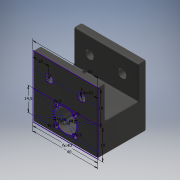
# Autodesk Inventor part: z_nut_holder
Saved by Autodesk Inventor 2018 (Build 220112000, 112)
## iProperties
Created: 2018-05-29
Part Number: z_nut_holder
Material: ABS Plastic
Document SubType Name: Modeling
Designer: Z. Deniz
Density: 1.06 g/cm^3
Appearance: Smooth - White
Author: Z. Deniz
Autodesk Inventor part; units mm, degrees
ref_plane "YZ Plane" through (0, 0, 0) normal (1, 0, 0) x (0, 1, 0)
ref_plane "XZ Plane" through (0, 0, 0) normal (0, 1, 0) x (-1, 0, 0)
ref_plane "XY Plane" through (0, 0, 0) normal (0, 0, 1) x (1, 0, 0)
sketch "Sketch1" plane through (0, 0, 0) normal (0, 1, 0) x (-1, 0, 0)
  circle A0 centre (0, 0) radius 7
  circle A1 centre (0, 0) radius 8 construction
  line L0 (0, 0) -> (5.6569, -5.6569) construction
  line L1 (0, 0) -> (8, 0) construction
  line L2 (0, 0) -> (-5.6569, -5.6569) construction
  line L3 (0, 0) -> (8, 0) construction
  line L4 (0, 0) -> (5.6569, 5.6569) construction
  line L5 (0, 0) -> (-5.6569, 5.6569) construction
  arc A2 (5.6319, 4.1571) -> (4.1571, 5.6319) centre (5.6569, 5.6569) ccw
  arc A3 (-4.1571, 5.6319) -> (-5.6319, 4.1571) centre (-5.6569, 5.6569) ccw
  arc A4 (-5.6319, -4.1571) -> (-4.1571, -5.6319) centre (-5.6569, -5.6569) ccw
  arc A5 (4.1571, -5.6319) -> (5.6319, -4.1571) centre (5.6569, -5.6569) ccw
  arc A6 (4.5962, 4.5962) -> (5.6319, 4.1571) centre (5.6569, 5.6569) ccw
  arc A7 (4.1571, 5.6319) -> (4.5962, 4.5962) centre (5.6569, 5.6569) ccw
  arc A8 (-4.5962, 4.5962) -> (-4.1571, 5.6319) centre (-5.6569, 5.6569) ccw
  arc A9 (-5.6319, 4.1571) -> (-4.5962, 4.5962) centre (-5.6569, 5.6569) ccw
  arc A10 (-4.5962, -4.5962) -> (-5.6319, -4.1571) centre (-5.6569, -5.6569) ccw
  arc A11 (-4.1571, -5.6319) -> (-4.5962, -4.5962) centre (-5.6569, -5.6569) ccw
  arc A12 (4.5962, -4.5962) -> (4.1571, -5.6319) centre (5.6569, -5.6569) ccw
  arc A13 (5.6319, -4.1571) -> (4.5962, -4.5962) centre (5.6569, -5.6569) ccw
  line L6 (-20, 7.25) -> (20, 7.25)
  line L7 (20, 7.25) -> (20, -7.25) construction
  line L8 (20, -7.25) -> (-20, -7.25) construction
  line L9 (-20, -7.25) -> (-20, 7.25) construction
  line L10 (-20, 7.25) -> (20, -7.25) construction
  line L11 (20, 7.25) -> (-20, -7.25) construction
  line L12 (20, 7.25) -> (-20, 7.25)
  line L13 (-20, 7.25) -> (-20, 27.25)
  line L14 (-20, 27.25) -> (20, 27.25)
  line L15 (20, 27.25) -> (20, 7.25)
  line L16 (20, 17.25) -> (-20, 17.25) construction
  circle A14 centre (10, 17.25) radius 2.5
  circle A15 centre (-10, 17.25) radius 2.5
  line L17 (20, 7.25) -> (-20, 7.25)
  line L18 (-20, 7.25) -> (-20, -10.75)
  line L19 (-20, -10.75) -> (20, -10.75)
  line L20 (20, -10.75) -> (20, 7.25)
  dimension "d0" = 14
  dimension "d1" = 16
  dimension "d2" = 45
  dimension "d3" = 135
  dimension "d4" = 3
  dimension "d5" = 3
  dimension "d6" = 3
  dimension "d7" = 3
  dimension "d9" = 14.5
  dimension "d10" = 20
  dimension "d11" = 40
  dimension "d14" = 5
  dimension "d15" = 5
  dimension "d16" = 10
  dimension "d17" = 10
  dimension "d22" = 18
  dimension "d23" = 40
  dimension "d24" = 40
  constraints: 42 end point, 28 point on circle, 15 centre point, 6 coincident, 6 parallel, 6 point on line, 5 horizontal, 5 perpendicular, 4 midpoint, 2 equal length, 10 other
  measures "d1" diameter of A1
  measures "d2" angle of L0 L1
  measures "d3" angle of L2 L3
  measures "d4" diameter of A2
  measures "d5" diameter of A3
  measures "d6" diameter of A4
  measures "d7" diameter of A5
  measures "d9" distance of L6.end L7.end
  measures "d10" distance of L12.end L13.end
  measures "d11" distance of L13.end L14.end
  measures "d14" diameter of A14
  measures "d15" diameter of A15
  measures "d16" distance from line of L15 A14.centre
  measures "d17" distance from line of L13 A15.centre
  measures "d22" distance of L18.end L17.end
  measures "d23" distance between parallel lines of L18 L20
  measures "d24" distance between parallel lines of L9 L20
extrude "Extrusion1" add sketch "Sketch1" along normal blind 5 contours L13 L14 L15 L6
extrude "Extrusion3" add sketch "Sketch1" along normal blind 25 contours L6 L20 L19 L18
sketch "Sketch3" plane through (0, 25, 0) normal (0, 1, 0) x (1, 0, 0)
  line L0 (20, -27.25) -> (20, -7.25) projected
  line L1 (-20, 10.75) -> (20, 10.75)
  line L2 (20, 10.75) -> (20, -27.25)
  line L3 (20, -27.25) -> (-20, -27.25)
  line L4 (-20, -27.25) -> (-20, 10.75)
  point P0 (0, 0)
  constraints: 8 end point, 2 parallel, 1 horizontal, 1 perpendicular
extrude "Extrusion4" add sketch "Sketch3" along normal blind 5
extrude "Extrusion5" cut sketch "Sketch1" along normal blind 30 contours A0 A13 A12 A11 A10 A9 A8 A7 A6 | A6 A7 A0 | A0 A2 | A5 A0 | A0 A12 A13 | A8 A9 A0 | A0 A3 | A4 A0 | A0 A10 A11 | A14 | A15
fillet "Fillet2" radius 1 24 edges at (-20, 15, 7.25) (0, 25, 7.25) (-20, 25, 17.25) (0, 25, 27.25) (-20, 27.5, 27.25) (0, 30, 27.25) (20, 27.5, 27.25) (20, 25, 17.25) (-20, 30, 8.25) (-20, 15, -10.75) (-20, 5, 17.25) (-20, 2.5, 27.25) (0, 5, 27.25) (0, 0, 27.25) (-20, 0, 8.25) (20, 0, 8.25) (20, 2.5, 27.25) (20, 15, 7.25) (0, 5, 7.25) (20, 5, 17.25) (20, 30, 8.25) (20, 15, -10.75) (0, 30, -10.75) (0, 0, -10.75)
equation "\"d4\" = d5"
equation "\"d6\" = d5"
equation "\"d7\" = d5"
equation "\"d11\" = d13"
equation "\"d17\" = d16"
equation "\"d24\" = d23"
equation "\"d13\" = 40"
body "Solid1"
